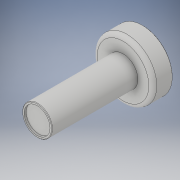
# Autodesk Inventor part: InfiniStix_066x
Saved by Autodesk Inventor 2019 (Build 230136000, 136)
## iProperties
Created: 2019-03-10
Part Number: InfiniStix_066x
Material: Generic
Document SubType Name: Modeling
Designer: Wilson Lab
Density: 1 g/cm^3
Appearance: Default
Author: Wilson Lab
Autodesk Inventor part; units mm, degrees
ref_plane "YZ Plane" through (0, 0, 0) normal (1, 0, 0) x (0, 1, 0)
ref_plane "XZ Plane" through (0, 0, 0) normal (0, 1, 0) x (-1, 0, 0)
ref_plane "XY Plane" through (0, 0, 0) normal (0, 0, 1) x (1, 0, 0)
sketch "Sketch1" plane through (0, 0, 0) normal (0, 0, 1) x (1, 0, 0)
  circle A0 centre (0, 0) radius 15
  dimension "d0" = 30
  constraints: 1 centre point, 1 coincident
  measures "d0" diameter of A0
extrude "Extrusion1" add sketch "Sketch1" along normal blind 10
sketch "Sketch2" plane through (0, 0, 10) normal (0, 0, 1) x (1, 0, 0)
  circle A0 centre (0, 0) radius 15 projected
  circle A1 centre (0, 0) radius 7.5
  dimension "d3" = 15
  constraints: 1 centre point, 1 coincident
  measures "d3" diameter of A1
extrude "Extrusion2" add sketch "Sketch2" along normal blind 43.2 contours A1
sketch "Sketch3" plane through (0, 0, 53.2) normal (0, 0, 1) x (1, 0, 0)
  circle A0 centre (0, 0) radius 7.5 projected
  circle A1 centre (0, 0) radius 6.5
  dimension "d6" = 1
  constraints: 1 centre point, 1 coincident
  measures "d6" radial gap between concentric circles of A1 A0
extrude "Extrusion3" cut sketch "Sketch3" against normal blind 1 contours A1
fillet "Fillet1" radius 2 1 edges at (-15, 0, 10)
chamfer "Chamfer1" distance 0.25 angle 45 1 edges at (-7.5, 0, 53.2)
chamfer "Chamfer2" distance 0.25 angle 45 1 edges at (-15, 0, 0)
body "Solid1"
